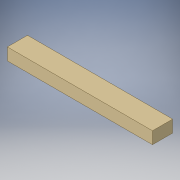
# Autodesk Inventor part: Rack and Pinion Wood Framing
Saved by Autodesk Inventor 2016 (Build 200138000, 138)
## iProperties
Created: 2016-04-02
Part Number: Rack and Pinion Wood Framing
Material: Generic
Document SubType Name: Modeling
Designer: amycroft3
Density: 1 g/cm^3
Appearance: Wheat
Author: amycroft3
Autodesk Inventor part; units mm, degrees
ref_plane "YZ Plane" through (0, 0, 0) normal (1, 0, 0) x (0, 1, 0)
ref_plane "XZ Plane" through (0, 0, 0) normal (0, 1, 0) x (-1, 0, 0)
ref_plane "XY Plane" through (0, 0, 0) normal (0, 0, 1) x (1, 0, 0)
sketch "Sketch1" plane through (0, 0, 0) normal (1, 0, 0) x (0, 1, 0)
  line L0 (-19.05, 31.75) -> (19.05, 31.75)
  line L1 (19.05, 31.75) -> (19.05, -31.75)
  line L2 (19.05, -31.75) -> (-19.05, -31.75)
  line L3 (-19.05, -31.75) -> (-19.05, 31.75)
  line L4 (-19.05, 31.75) -> (19.05, -31.75) construction
  line L5 (19.05, 31.75) -> (-19.05, -31.75) construction
  point P0 (0, 0)
  dimension "d0" = 38.1
  dimension "d1" = 63.5
  constraints: 12 end point, 2 midpoint, 2 parallel, 1 horizontal, 1 perpendicular
  measures "d0" distance of L1.end L2.end
  measures "d1" distance of L0.end L1.end
extrude "Extrusion1" add sketch "Sketch1" along normal blind 457.2
body "Solid1"
